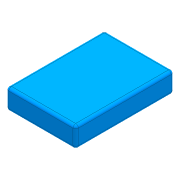
# Autodesk Inventor part: ServoBattery
Saved by Autodesk Inventor 2018 (Build 220112000, 112)
## iProperties
Created: 2018-10-15
Part Number: ServoBattery
Material: Generic
Document SubType Name: Modeling
Designer: Vulnic
Density: 2.58162 g/cm^3
Appearance: Default
Mass: 141 g
Surface Area: 105.556 cm^2
Volume: 54.6169 cm^3
Author: Vulnic
Autodesk Inventor part; units mm, degrees
ref_plane "YZ Plane" through (0, 0, 0) normal (1, 0, 0) x (0, 1, 0)
ref_plane "XZ Plane" through (0, 0, 0) normal (0, 1, 0) x (-1, 0, 0)
ref_plane "XY Plane" through (0, 0, 0) normal (0, 0, 1) x (1, 0, 0)
sketch "Sketch1" plane through (0, 0, 0) normal (0, 0, 1) x (1, 0, 0)
  line L0 (-25.5, -36) -> (25.5, -36)
  line L1 (25.5, -36) -> (25.5, 36)
  line L2 (25.5, 36) -> (-25.5, 36)
  line L3 (-25.5, 36) -> (-25.5, -36)
  line L4 (-25.5, -36) -> (25.5, 36) construction
  line L5 (25.5, -36) -> (-25.5, 36) construction
  point P0 (0, 0)
  dimension "d0" = 51
  dimension "d1" = 72
  constraints: 12 end point, 2 midpoint, 2 parallel, 1 horizontal, 1 perpendicular
  measures "d0" distance of L1.end L2.end
  measures "d1" distance of L0.end L1.end
extrude "Extrusion1" add sketch "Sketch1" along normal blind 15
fillet "Fillet1" radius 2 12 edges at (25.5, 0, 0) (0, 36, 0) (25.5, 36, 7.5) (0, 36, 15) (25.5, 0, 15) (25.5, -36, 7.5) (0, -36, 15) (0, -36, 0) (-25.5, -36, 7.5) (-25.5, 0, 15) (-25.5, 0, 0) (-25.5, 36, 7.5)
body "Solid1"
